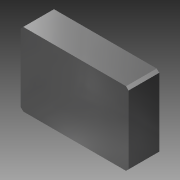
# Autodesk Inventor part: Rasp
Saved by Autodesk Inventor 2014 SP1 (Build 180222100, 222)
## iProperties
Created: 2017-02-18
Part Number: Rasp
Material: Plástico PBT
Document SubType Name: Modeling
Designer: Tizon
Density: 1.31 g/cm^3
Appearance: Cromo - Negro Pulido
Mass: 151.775 g
Surface Area: 176.872 cm^2
Volume: 115.859 cm^3
Author: Tizon
Autodesk Inventor part; units mm, degrees
ref_plane "YZ Plane" through (0, 0, 0) normal (1, 0, 0) x (0, 1, 0)
ref_plane "XZ Plane" through (0, 0, 0) normal (0, 1, 0) x (-1, 0, 0)
ref_plane "XY Plane" through (0, 0, 0) normal (0, 0, 1) x (1, 0, 0)
sketch "Boceto1" plane through (0, 0, 0) normal (0, 1, 0) x (-1, 0, 0)
  line L0 (88, 0) -> (0, 0)
  line L1 (0, 0) -> (0, 58.5)
  line L2 (0, 58.5) -> (88, 58.5)
  line L3 (88, 58.5) -> (88, 0)
  dimension "d0" = 58.5
  dimension "d1" = 88
  constraints: 8 end point, 2 parallel, 1 coincident, 1 horizontal, 1 perpendicular
  measures "d0" distance of L0.end L1.end
  measures "d1" distance of L1.end L2.end
extrude "Extrusión1" add sketch "Boceto1" along normal blind 24.5
sketch "Boceto2" plane through (0, 24.5, 0) normal (0, 1, 0) x (1, 0, 0)
  line L0 (0, 0) -> (-88, 0) projected
  line L1 (-88, 0) -> (-88, -58.5) projected
  line L2 (-88, -58.5) -> (0, -58.5) projected
  line L3 (0, -58.5) -> (0, 0) projected
  line L4 (-36, -58.5) -> (0, -58.5)
  line L5 (-36.5, -58.5) -> (-38.5, -58.5)
  line L6 (-39, -58) -> (-39, -40)
  line L7 (-38.5, -39.5) -> (-36.5, -39.5)
  line L8 (-36, -40) -> (-36, -58)
  line L9 (0, 0) -> (-22.5, 0)
  line L10 (-22.5, 0) -> (-82.5, 0)
  line L11 (-82.5, 0) -> (-82.5, -8)
  line L12 (-80.5, -10) -> (-24.5, -10)
  line L13 (-22.5, -8) -> (-22.5, 0)
  arc A0 (-24.5, -10) -> (-22.5, -8) centre (-24.5, -8) ccw
  arc A1 (-82.5, -8) -> (-80.5, -10) centre (-80.5, -8) ccw
  arc A2 (-38.5, -39.5) -> (-39, -40) centre (-38.5, -40) ccw
  arc A3 (-36, -40) -> (-36.5, -39.5) centre (-36.5, -40) ccw
  arc A4 (-36.5, -58.5) -> (-36, -58) centre (-36.5, -58) ccw
  arc A5 (-39, -58) -> (-38.5, -58.5) centre (-38.5, -58) ccw
  line L14 (0, 0) -> (-86, 0)
  line L15 (-86, 0) -> (-86, -58.5)
  line L16 (-86, -58.5) -> (0, -58.5)
  line L17 (0, -58.5) -> (0, 0)
  line L18 (-38.6961, -58.4599) -> (-36.3039, -58.4599)
  point P0 (-39, -39.5)
  point P1 (-36, -39.5)
  dimension "d4" = 36
  dimension "d5" = 19
  dimension "d6" = 3
  dimension "d7" = 22.5
  dimension "d8" = 2
  dimension "d9" = 0.5
  dimension "d10" = 56
  dimension "d11" = 88
  dimension "d12" = 58.5
  dimension "d13" = 86
  dimension "d14" = 10
  dimension "d15" = 2.3923
  constraints: 30 end point, 14 point on circle, 12 tangent, 10 point on line, 6 centre point, 5 parallel, 4 equal radius, 4 perpendicular, 2 collinear, 2 horizontal
  measures "d4" distance of L4.start L2.end
  measures "d5" distance of point (-36, -39.5) L4.start
  measures "d6" distance of point (-39, -39.5) point (-36, -39.5)
  measures "d7" distance of L0.start L9.end
  measures "d8" radius of A0
  measures "d9" radius of A2
  measures "d10" distance of L12.start L12.end
  measures "d11" distance of L1.end L2.end
  measures "d12" distance of L0.end L1.end
  measures "d13" distance of L0.start L14.end
  measures "d14" distance between parallel lines of L12 L14
  measures "d15" distance of L18.start L18.end
extrude "Extrusión2" cut sketch "Boceto2" against normal blind 11 contours L13 A0 L12 A1 L11 L0 | L15 L2 L1 L0 | L18 A5 L6 A2 L7 A3 L8 A4
sketch "Boceto3" plane through (0, 24.5, 0) normal (0, 1, 0) x (1, 0, 0)
  line L0 (-86, 0) -> (-86, -58.5) projected
  line L1 (-86, -58.5) -> (0, -58.5) projected
  line L2 (0, -58.5) -> (0, 0) projected
  line L3 (0, 0) -> (-22.5, 0) projected
  line L4 (-22.5, 0) -> (-22.5, -8) projected
  arc A0 (-24.5, -10) -> (-22.5, -8) centre (-24.5, -8) ccw projected
  line L5 (-24.5, -10) -> (-80.5, -10) projected
  arc A1 (-82.5, -8) -> (-80.5, -10) centre (-80.5, -8) ccw projected
  line L6 (-82.5, -8) -> (-82.5, 0) projected
  line L7 (-82.5, 0) -> (-86, 0) projected
  line L8 (-39, -58) -> (-39, -40) projected
  arc A2 (-38.5, -39.5) -> (-39, -40) centre (-38.5, -40) ccw projected
  line L9 (-38.5, -39.5) -> (-36.5, -39.5) projected
  arc A3 (-36, -40) -> (-36.5, -39.5) centre (-36.5, -40) ccw projected
  line L10 (-36, -40) -> (-36, -58) projected
  arc A4 (-36.3039, -58.4599) -> (-36, -58) centre (-36.5, -58) ccw projected
  line L11 (-36.3039, -58.4599) -> (-38.6961, -58.4599) projected
  arc A5 (-39, -58) -> (-38.6961, -58.4599) centre (-38.5, -58) ccw projected
sketch "Boceto4" plane through (0, 13.5, 0) normal (0, 1, 0) x (1, 0, 0)
  line L0 (-88, -58.5) -> (-88, 0) projected
  line L1 (-86, -58.5) -> (-88, -58.5) projected
  line L2 (-88, 0) -> (-86, 0)
  line L3 (-86, 0) -> (-86, -58.5)
  line L4 (-86, -58.5) -> (-88, -58.5)
  line L5 (-88, -58.5) -> (-88, 0)
  point P0 (0, 0)
  constraints: 8 end point, 2 parallel, 1 horizontal, 1 perpendicular
extrude "Extrusión3" cut sketch "Boceto4" against normal blind 50
chamfer "Chaflán1" distance 2 angle 45 1 edges at (0, 12.25, 58.5)
chamfer "Chaflán2" distance 2 angle 45 1 edges at (0, 12.25, 0)
chamfer "Chaflán3" distance 2 angle 45 1 edges at (-86, 12.25, 58.5)
chamfer "Chaflán4" distance 2 angle 45 1 edges at (-86, 12.25, 0)
